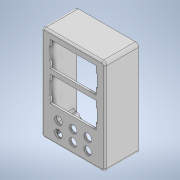
# Autodesk Inventor part: front_case
Saved by Autodesk Inventor 2022.1 (Build 261234020, 234B)
## iProperties
Created: 2022-02-06
Part Number: front_case
Material: Polylactic Acid (PLA)
Document SubType Name: Modeling
Designer: kee
Mass: 129.863 g
Surface Area: 612.227 cm^2
Volume: 103.891 cm^3
Density: 1.25 g/cm^3
Appearance: Default
Author: kee
Autodesk Inventor part; units mm, degrees
ref_plane "YZ Plane" through (0, 0, 0) normal (1, 0, 0) x (0, 1, 0)
ref_plane "XZ Plane" through (0, 0, 0) normal (0, 1, 0) x (-1, 0, 0)
ref_plane "XY Plane" through (0, 0, 0) normal (0, 0, 1) x (1, 0, 0)
sketch "Sketch1" plane through (0, 0, 0) normal (0, 0, 1) x (1, 0, 0)
  line L0 (-45, 75) -> (45, 75)
  line L1 (50, 70) -> (50, -70)
  line L2 (45, -75) -> (-45, -75)
  line L3 (-50, -70) -> (-50, 70)
  arc A0 (-45, 75) -> (-50, 70) centre (-45, 70) ccw
  arc A1 (50, 70) -> (45, 75) centre (45, 70) ccw
  arc A2 (-50, -70) -> (-45, -75) centre (-45, -70) ccw
  arc A3 (45, -75) -> (50, -70) centre (45, -70) ccw
  point P0 (0, 0)
  point P1 (-50, 75)
  point P2 (50, -75)
  point P3 (50, 75)
  point P4 (-50, -75)
  point P5 (50, 0)
  dimension "d3" = 100
  dimension "d4" = 50
  dimension "d5" = 150
  dimension "d6" = 75
  dimension "d37" = 5
  dimension "d125" = 90
  dimension "d126" = 140
  constraints: 8 end point, 8 point on circle, 8 point on line, 8 tangent, 4 centre point, 3 equal radius, 2 parallel, 1 horizontal, 1 midpoint, 1 perpendicular
  measures "d3" distance between parallel lines of L1 L3
  measures "d4" distance of point (50, 0) point (0, 0)
  measures "d5" distance between parallel lines of L2 L0
  measures "d6" distance from line of L2 point (0, 0)
  measures "d37" radius of A0
  measures "d125" distance of A0.centre A1.centre
  measures "d126" distance of A3.centre A1.centre
extrude "Extrusion1" add sketch "Sketch1" along normal blind 3
sketch "Sketch2" plane through (0, 0, 3) normal (0, 0, 1) x (1, 0, 0)
  circle A0 centre (-23, -40) radius 6
  circle A1 centre (-23, -58) radius 6
  circle A2 centre (0, -40) radius 6
  circle A3 centre (0, -58) radius 6
  circle A4 centre (23, -40) radius 6
  circle A5 centre (23, -58) radius 6
  line L0 (-45, -75) -> (45, -75) projected
  line L1 (-36, 17) -> (36, 17)
  line L2 (36, 17) -> (36, 7)
  line L3 (36, 7) -> (38, 7)
  line L4 (38, 7) -> (38, -13)
  line L5 (38, -13) -> (36, -13)
  line L6 (36, -13) -> (36, -23)
  line L7 (36, -23) -> (-36, -23)
  line L8 (-36, -23) -> (-36, -13)
  line L9 (-36, -13) -> (-38, -13)
  line L10 (-38, -13) -> (-38, 7)
  line L11 (-38, 7) -> (-36, 7)
  line L12 (-36, 17) -> (-36, 7)
  line L13 (-36, 64.5) -> (36, 64.5)
  line L14 (36, 64.5) -> (36, 54.5)
  line L15 (36, 54.5) -> (38, 54.5)
  line L16 (38, 54.5) -> (38, 34.5)
  line L17 (38, 34.5) -> (36, 34.5)
  line L18 (36, 34.5) -> (36, 24.5)
  line L19 (36, 24.5) -> (-36, 24.5)
  line L20 (-36, 24.5) -> (-36, 34.5)
  line L21 (-36, 34.5) -> (-38, 34.5)
  line L22 (-38, 34.5) -> (-38, 54.5)
  line L23 (-38, 54.5) -> (-36, 54.5)
  line L24 (-36, 64.5) -> (-36, 54.5)
  point P0 (-50, -70)
  point P1 (50, -70)
  point P2 (0, 0)
  point P3 (0, 47.5)
  dimension "d7" = 12
  dimension "d8" = 12
  dimension "d9" = 12
  dimension "d10" = 12
  dimension "d11" = 12
  dimension "d12" = 12
  dimension "d13" = 23
  dimension "d14" = 23
  dimension "d15" = 18
  dimension "d18" = 72
  dimension "d19" = 36
  dimension "d20" = 40
  dimension "d21" = 10
  dimension "d22" = 10
  dimension "d23" = 2
  dimension "d24" = 2
  dimension "d27" = 23
  dimension "d28" = 72
  dimension "d29" = 36
  dimension "d30" = 40
  dimension "d31" = 10
  dimension "d32" = 10
  dimension "d33" = 2
  dimension "d34" = 2
  dimension "d35" = 23
  dimension "d36" = 7.5
  dimension "d100" = 52
  dimension "d101" = 17
  constraints: 48 end point, 14 perpendicular, 14 point on line, 6 centre point, 4 horizontal alignment, 4 vertical alignment, 2 horizontal, 2 vertical, 1 other
  measures "d7" diameter of A0
  measures "d8" diameter of A1
  measures "d9" diameter of A2
  measures "d10" diameter of A3
  measures "d11" diameter of A4
  measures "d12" diameter of A5
  measures "d13" distance of A2.centre A0.centre
  measures "d14" distance of A4.centre A2.centre
  measures "d15" distance of A5.centre A4.centre
  measures "d18" distance of L1.start L1.end
  measures "d19" distance from line of L2 point (0, 0)
  measures "d20" distance between parallel lines of L7 L1
  measures "d21" distance of L1.end L2.end
  measures "d22" distance of L5.end L6.end
  measures "d23" distance between parallel lines of L4 L6
  measures "d24" distance between parallel lines of L10 L8
  measures "d27" distance from line of L7 point (0, 0)
  measures "d28" distance of L24.start L14.start
  measures "d29" distance from line of L14 point (0, 47.5)
  measures "d30" distance between parallel lines of L19 L13
  measures "d31" distance of L14.start L15.start
  measures "d32" distance of L18.start L19.start
  measures "d33" distance between parallel lines of L16 L18
  measures "d34" distance between parallel lines of L22 L20
  measures "d35" distance from line of L19 point (0, 47.5)
  measures "d36" distance between parallel lines of L1 L19
  measures "d100" vertical distance of point (45, -75) L6.end
  measures "d101" distance from line of L7 A4.centre
extrude "Extrusion2" cut sketch "Sketch2" against normal up to next
sketch "Sketch5" plane through (0, 0, 0) normal (0, 0, -1) x (-1, 0, 0)
  circle A0 centre (23, -40) radius 6 projected
  circle A1 centre (0, -58) radius 6 projected
  circle A2 centre (23, -58) radius 6 projected
  line L0 (38, 7) -> (38, -13) projected
  line L1 (38, -13) -> (36, -13) projected
  line L2 (36, -13) -> (36, -23) projected
  line L3 (36, -23) -> (-36, -23) projected
  line L4 (-36, -23) -> (-36, -13) projected
  line L5 (-36, -13) -> (-38, -13) projected
  line L6 (-38, -13) -> (-38, 7) projected
  line L7 (-38, 7) -> (-36, 7) projected
  line L8 (-36, 7) -> (-36, 17) projected
  line L9 (-36, 17) -> (36, 17) projected
  line L10 (36, 17) -> (36, 7) projected
  line L11 (36, 7) -> (38, 7) projected
  circle A3 centre (0, -40) radius 6 projected
  circle A4 centre (-23, -58) radius 6 projected
  circle A5 centre (-23, -40) radius 6 projected
  line L12 (38, 54.5) -> (38, 34.5) projected
  line L13 (38, 34.5) -> (36, 34.5) projected
  line L14 (36, 34.5) -> (36, 24.5) projected
  line L15 (36, 24.5) -> (-36, 24.5) projected
  line L16 (-36, 24.5) -> (-36, 34.5) projected
  line L17 (-36, 34.5) -> (-38, 34.5) projected
  line L18 (-38, 34.5) -> (-38, 54.5) projected
  line L19 (-38, 54.5) -> (-36, 54.5) projected
  line L20 (-36, 54.5) -> (-36, 64.5) projected
  line L21 (-36, 64.5) -> (36, 64.5) projected
  line L22 (36, 64.5) -> (36, 54.5) projected
  line L23 (36, 54.5) -> (38, 54.5) projected
  line L24 (45, -75) -> (-45, -75) projected
  arc A6 (45, -75) -> (50, -70) centre (45, -70) ccw projected
  line L25 (50, 70) -> (50, -70) projected
  arc A7 (50, 70) -> (45, 75) centre (45, 70) ccw projected
  line L26 (-45, 75) -> (45, 75) projected
  arc A8 (-45, 75) -> (-50, 70) centre (-45, 70) ccw projected
  line L27 (-50, -70) -> (-50, 70) projected
  arc A9 (-50, -70) -> (-45, -75) centre (-45, -70) ccw projected
  arc A10 (47, 70) -> (45, 72) centre (45, 70) ccw
  line L28 (47, 70) -> (47, -70)
  arc A11 (45, -72) -> (47, -70) centre (45, -70) ccw
  line L29 (45, -72) -> (-45, -72)
  arc A12 (-47, -70) -> (-45, -72) centre (-45, -70) ccw
  line L30 (-47, -70) -> (-47, 70)
  arc A13 (-45, 72) -> (-47, 70) centre (-45, 70) ccw
  line L31 (-45, 72) -> (45, 72)
  line L32 (-45, 75) -> (45, 75)
  arc A14 (50, 70) -> (45, 75) centre (45, 70) ccw
  line L33 (50, 70) -> (50, -70)
  arc A15 (45, -75) -> (50, -70) centre (45, -70) ccw
  line L34 (45, -75) -> (-45, -75)
  arc A16 (-50, -70) -> (-45, -75) centre (-45, -70) ccw
  line L35 (-50, -70) -> (-50, 70)
  arc A17 (-45, 75) -> (-50, 70) centre (-45, 70) ccw
  line L36 (-116.3396, 0) -> (109.1655, 0) construction
  line L37 (0, 86.6309) -> (0, -88.1774) construction
  line L38 (-47, 62) -> (-42, 62)
  line L39 (-37, 67) -> (-37, 72)
  arc A18 (-42, 62) -> (-37, 67) centre (-42, 67) ccw
  line L40 (47, 62) -> (42, 62)
  line L41 (37, 67) -> (37, 72)
  arc A19 (37, 67) -> (42, 62) centre (42, 67) ccw
  line L42 (37, -72) -> (37, -67)
  line L43 (42, -62) -> (47, -62)
  arc A20 (42, -62) -> (37, -67) centre (42, -67) ccw
  line L44 (-37, -72) -> (-37, -67)
  line L45 (-42, -62) -> (-47, -62)
  arc A21 (-37, -67) -> (-42, -62) centre (-42, -67) ccw
  point P0 (0, 0)
  point P1 (-37, 62)
  point P2 (37, 62)
  point P3 (37, -62)
  point P4 (-37, -62)
  dimension "d38" = 3
  dimension "d103" = 10
  dimension "d104" = 10
  dimension "d105" = 5
  dimension "d108" = 10
  dimension "d109" = 10
  dimension "d110" = 5
  dimension "d111" = 10
  dimension "d112" = 10
  dimension "d113" = 5
  dimension "d114" = 10
  dimension "d115" = 10
  dimension "d116" = 5
  dimension "d127" = 84
  dimension "d128" = 134
  constraints: 36 end point, 24 point on circle, 18 point on line, 13 tangent, 12 centre point, 5 perpendicular, 4 coincident, 4 horizontal, 4 vertical, 7 other
  measures "d38" distance between parallel lines of L26 L31
  measures "d103" distance of L38.start point (-37, 62)
  measures "d104" distance of point (-37, 62) L39.end
  measures "d105" radius of A18
  measures "d108" distance of L40.start point (37, 62)
  measures "d109" distance of point (37, 62) L41.end
  measures "d110" radius of A19
  measures "d111" distance of L42.start point (37, -62)
  measures "d112" distance of point (37, -62) L43.end
  measures "d113" radius of A20
  measures "d114" distance of L44.start point (-37, -62)
  measures "d115" distance of point (-37, -62) L45.end
  measures "d116" radius of A21
  measures "d127" distance of A19.centre A18.centre
  measures "d128" distance of A20.centre A19.centre
extrude "Extrusion13" add sketch "Sketch5" along normal blind 50 contours L24 A9 L27 A8 L26 A7 L25 A6 | L28 L40 A19 L41 L31 A10 | L28 A11 L29 L42 A20 L43 | L39 A18 L38 L30 A13 L31 | L29 A12 L30 L45 A21 L44
sketch "Sketch17" plane through (0, 0, -50) normal (0, 0, -1) x (-1, 0, 0)
  line L0 (-45, -75) -> (45, -75) projected
  arc A0 (45, -75) -> (50, -70) centre (45, -70) ccw projected
  line L1 (50, -70) -> (50, 70) projected
  arc A1 (50, 70) -> (45, 75) centre (45, 70) ccw projected
  line L2 (45, 75) -> (-45, 75) projected
  arc A2 (-45, 75) -> (-50, 70) centre (-45, 70) ccw projected
  line L3 (-50, 70) -> (-50, -70) projected
  arc A3 (-50, -70) -> (-45, -75) centre (-45, -70) ccw projected
  line L4 (37, 72) -> (37, 67) projected
  arc A4 (37, 67) -> (42, 62) centre (42, 67) ccw projected
  line L5 (42, 62) -> (47, 62) projected
  line L6 (47, 62) -> (47, -62) projected
  line L7 (47, -62) -> (42, -62) projected
  arc A5 (42, -62) -> (37, -67) centre (42, -67) ccw projected
  line L8 (37, -67) -> (37, -72) projected
  line L9 (37, -72) -> (-37, -72) projected
  line L10 (-37, -72) -> (-37, -67) projected
  arc A6 (-37, -67) -> (-42, -62) centre (-42, -67) ccw projected
  line L11 (-42, -62) -> (-47, -62) projected
  line L12 (-47, -62) -> (-47, 62) projected
  line L13 (-47, 62) -> (-42, 62) projected
  arc A7 (-42, 62) -> (-37, 67) centre (-42, 67) ccw projected
  line L14 (-37, 67) -> (-37, 72) projected
  line L15 (-37, 72) -> (37, 72) projected
  line L16 (-42, 72) -> (42, 72)
  line L17 (47, 67) -> (47, -67)
  line L18 (42, -72) -> (-42, -72)
  line L19 (-47, -67) -> (-47, 67)
  arc A8 (-42, 72) -> (-47, 67) centre (-42, 67) ccw
  arc A9 (47, 67) -> (42, 72) centre (42, 67) ccw
  arc A10 (42, -72) -> (47, -67) centre (42, -67) ccw
  arc A11 (-47, -67) -> (-42, -72) centre (-42, -67) ccw
  point P0 (0, 0)
  point P1 (-47, 72)
  point P2 (-47, 62)
  dimension "d117" = 5
  constraints: 8 end point, 8 point on circle, 8 tangent, 4 centre point, 3 equal radius, 3 point on line, 2 parallel, 1 horizontal, 1 perpendicular
  measures "d117" radius of A8
extrude "Extrusion14" cut sketch "Sketch17" against normal blind 5 contours L16 A9 L17 L5 A4 L4 | L4 A4 L5 L6 L7 A5 L8 L9 L10 A6 L11 L12 L13 A7 L14 L15 | L14 A7 L13 L19 A8 L16 | L17 A10 L18 L8 A5 L7 | L11 A6 L10 L18 A11 L19
sketch "Sketch18" plane through (-45, -75, 3) normal (0, -1, 0) x (1, 0, 0)
  line L0 (3, -53) -> (87, -53) projected
  line L1 (85, -53) -> (5, -53)
  line L2 (5, -53) -> (5, -10)
  line L3 (5, -10) -> (85, -10)
  line L4 (85, -10) -> (85, -53)
  line L5 (0, 0) -> (90, 0) projected
  line L6 (45, -65.8831) -> (45, 5.9535) construction
  point P0 (45, -3)
  point P1 (45, 0)
  point P2 (5, -53)
  dimension "d120" = 10
  dimension "d121" = 80
  dimension "d122" = 40
  constraints: 10 end point, 2 parallel, 2 point on line, 1 horizontal, 1 midpoint, 1 perpendicular, 1 vertical
  measures "d120" distance between parallel lines of L5 L3
  measures "d121" distance between parallel lines of L2 L4
  measures "d122" distance between parallel lines of L2 L6
extrude "Extrusion15" cut sketch "Sketch18" against normal up to surface (3 mm away)
fillet "Fillet1" radius 3 2 edges at (40, -73.5, -7) (-40, -73.5, -7)
sketch "Sketch19" plane through (0, 0, -45) normal (0, 0, -1) x (-1, 0, 0)
  line L0 (-42, 62) -> (-47, 62) construction
  arc A0 (-42, 62) -> (-37, 67) centre (-42, 67) ccw construction
  line L1 (-37, 72) -> (-37, 67) construction
  line L2 (-42, 72) -> (-37, 72) construction
  arc A1 (-42, 72) -> (-47, 67) centre (-42, 67) ccw construction
  line L3 (-47, 62) -> (-47, 67) construction
  line L4 (47, 62) -> (42, 62) construction
  line L5 (47, 67) -> (47, 62) construction
  arc A2 (47, 67) -> (42, 72) centre (42, 67) ccw construction
  line L6 (37, 72) -> (42, 72) construction
  line L7 (37, 67) -> (37, 72) construction
  arc A3 (37, 67) -> (42, 62) centre (42, 67) ccw construction
  line L8 (37, -72) -> (37, -67) construction
  line L9 (40, -72) -> (37, -72) construction
  line L10 (42, -72) -> (40, -72) construction
  arc A4 (42, -72) -> (47, -67) centre (42, -67) ccw construction
  line L11 (47, -62) -> (47, -67) construction
  line L12 (42, -62) -> (47, -62) construction
  arc A5 (42, -62) -> (37, -67) centre (42, -67) ccw construction
  line L13 (-37, -67) -> (-37, -72) construction
  arc A6 (-37, -67) -> (-42, -62) centre (-42, -67) ccw construction
  line L14 (-47, -62) -> (-42, -62) construction
  line L15 (-47, -67) -> (-47, -62) construction
  arc A7 (-47, -67) -> (-42, -72) centre (-42, -67) ccw construction
  line L16 (-40, -72) -> (-42, -72) construction
  line L17 (-37, -72) -> (-40, -72) construction
  point P0 (0, 0)
hole "Hole1" at (42, 67, -45) at (-42, 67, -45) at (-42, -67, -45) at (42, -67, -45) direction (0, 0, 1) diameter 3 depth 15 tip angle 118
fillet "Fillet2" radius 3 29 edges at (48.5355, 73.5355, 3) (0, 75, 3) (-48.5355, 73.5355, 3) (-50, 0, 3) (-48.5355, -73.5355, 3) (0, -75, 3) (48.5355, -73.5355, 3) (50, 0, 3) (47, 62, -22.5) (37, 72, -22.5) (-47, 62, -22.5) (-37, 72, -22.5) (-47, -62, -22.5) (47, -62, -22.5) (47, 0, 0) (37, -69.5, 0) (44.5, -62, 0) (38.4645, -63.4645, 0) (-38.4645, -63.4645, 0) (-44.5, -62, 0) (-37, -69.5, 0) (0, -72, 0) (0, 72, 0) (38.4645, 63.4645, 0) (44.5, 62, 0) (37, 69.5, 0) (-38.4645, 63.4645, 0) (-44.5, 62, 0) (-37, 69.5, 0)
equation "\"d4\" = 0.5 * d3"
equation "\"d6\" = 0.5 * d5"
equation "\"d14\" = d13"
equation "\"d19\" = 0.5 * d18"
equation "\"d29\" = 0.5 * d28"
body "Solid1"
